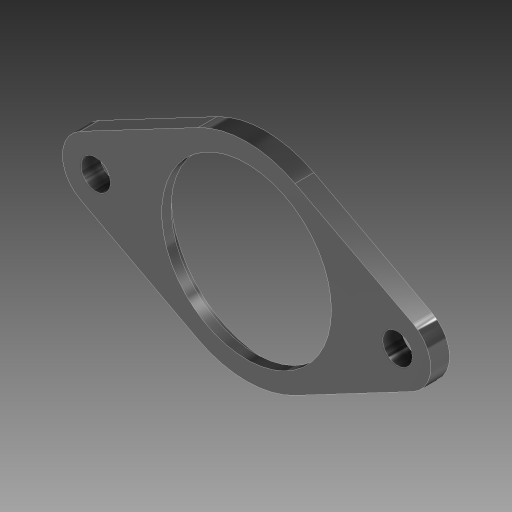
# Autodesk Inventor part: Thriftybot Bearing Hat (TTB-0059)
Saved by Autodesk Inventor 2023 (Build 270158030, 158C)
## iProperties
Created: 2022-12-19
Part Number: Thriftybot Bearing Hat (TTB-0059)
Material: Aluminum 6061
Document SubType Name: Modeling
Designer: Max Boord
Density: 2.7 g/cm^3
Appearance: Glazed - Black
Author: Max Boord
Autodesk Inventor part; units mm, degrees
ref_plane "YZ Plane" through (0, 0, 0) normal (1, 0, 0) x (0, 1, 0)
ref_plane "XZ Plane" through (0, 0, 0) normal (0, 1, 0) x (-1, 0, 0)
ref_plane "XY Plane" through (0, 0, 0) normal (0, 0, 1) x (1, 0, 0)
sketch "Sketch1" plane through (0, 0, 0) normal (0, 0, 1) x (1, 0, 0)
  circle A0 centre (0, 0) radius 14.2875
  circle A1 centre (0, 0) radius 15.875
  line L0 (-28.0155, -4.9525) -> (-8.155, -15.4413)
  line L1 (28.0155, -4.9525) -> (8.155, -15.4413)
  line L2 (-8.155, 15.4413) -> (-28.0155, 4.9525)
  line L3 (8.155, 15.4413) -> (28.0155, 4.9525)
  arc A2 (8.155, 15.4413) -> (-8.155, 15.4413) centre (0, 0) ccw
  arc A3 (-8.155, -15.4413) -> (8.155, -15.4413) centre (0, 0) ccw
  arc A4 (-28.0155, 4.9525) -> (-28.0155, -4.9525) centre (-25.4, 0) ccw
  arc A5 (28.0155, -4.9525) -> (28.0155, 4.9525) centre (25.4, 0) ccw
  circle A6 centre (-25.4, 0) radius 2.4892
  circle A7 centre (25.4, 0) radius 2.4892
  dimension "d0" = 28.575
  dimension "d2" = 31.75
  dimension "d3" = 34.925
  dimension "d4" = 4.9784
  dimension "d5" = 50.8
  dimension "d6" = 11.2014
  constraints: 8 centre point, 8 end point, 8 point on circle, 8 tangent, 3 coincident, 3 equal length, 2 equal radius, 2 horizontal alignment
  measures "d0" diameter of A0
  measures "d2" diameter of A1
  measures "d3" diameter of A2
  measures "d4" diameter of A6
  measures "d5" distance of A5.centre A4.centre
  measures "d6" diameter of A4
extrude "Extrusion1" add sketch "Sketch1" along normal mid plane 3.175 contours A1 | A4 L2 A2 L3 A5 L1 A3 L0
extrude "Extrusion2" cut sketch "Sketch1" against normal blind 1.5875 contours A1
body "Solid1"
